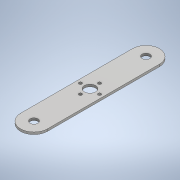
# Autodesk Inventor part: hip_link_motor
Saved by Autodesk Inventor 2022 (Build 260153000, 153)
## iProperties
Category: リンク
Created: 2016-08-23
Part Number: hip_link_motor
Material: GFRP
Document SubType Name: Modeling
Designer: hiro
Density: 1.75 g/cm^3
Appearance: 滑らか - 淡い灰色
Mass: 6.98824 g
Surface Area: 46.6416 cm^2
Volume: 3.99328 cm^3
Author: hiro
Autodesk Inventor part; units mm, degrees
ref_plane "YZ Plane" through (0, 0, 0) normal (1, 0, 0) x (0, 1, 0)
ref_plane "XZ Plane" through (0, 0, 0) normal (0, 1, 0) x (-1, 0, 0)
ref_plane "XY Plane" through (0, 0, 0) normal (0, 0, 1) x (1, 0, 0)
sketch "スケッチ1" plane through (0, 0, 0) normal (0, 0, 1) x (1, 0, 0)
  line L0 (24, 0) -> (24, 100)
  line L1 (0, 100) -> (0, 0)
  line L2 (12, 100) -> (12, 0) construction
  arc A0 (24, 100) -> (0, 100) centre (12, 100) ccw
  arc A1 (0, 0) -> (24, 0) centre (12, 0) ccw
  circle A2 centre (12, 0) radius 3.5
  circle A3 centre (12, 100) radius 3.5
  circle A4 centre (12, 50) radius 5
  dimension "d35" = 24
  dimension "d36" = 100
  dimension "d37" = 7
  dimension "d38" = 7
  dimension "d41" = 10
  constraints: 6 end point, 5 centre point, 4 coincident, 4 point on circle, 2 horizontal alignment, 1 midpoint, 1 parallel, 1 vertical, 1 vertical alignment, 1 other
  measures "d35" distance of L0.start L1.end
  measures "d36" distance of L1.start L1.end
  measures "d37" diameter of A2
  measures "d38" diameter of A3
  measures "d41" diameter of A4
extrude "押し出し1" add sketch "スケッチ1" along normal blind 2
sketch "スケッチ3" plane through (0, 0, 2) normal (0, 0, 1) x (1, 0, 0)
  circle A0 centre (12, 0) radius 3.5 projected
  circle A1 centre (12, 100) radius 3.5 projected
  circle A2 centre (12, 50) radius 5 projected
  arc A3 (24, 100) -> (0, 100) centre (12, 100) ccw projected
  line L0 (0, 100) -> (0, 0) projected
  arc A4 (0, 0) -> (24, 0) centre (12, 0) ccw projected
  line L1 (24, 0) -> (24, 100) projected
  line L2 (12, 50) -> (24, 50) construction
  line L3 (24, 0) -> (24, 100) projected
  point P0 (20.5, 50)
  point P1 (12, 58.5)
  point P2 (3.5, 50)
  point P3 (12, 41.5)
  dimension "d42" = 8.5
  dimension "d45" = 360
  constraints: 2 end point, 1 midpoint, 1 point on line, 5 other
  measures "d42" distance of point (20.5, 50) L2.start
hole "穴1" at (20.5, 50, 2) at (12, 58.5, 2) at (3.5, 50, 2) at (12, 41.5, 2) direction (0, 0, -1) diameter 2.8 end through all
